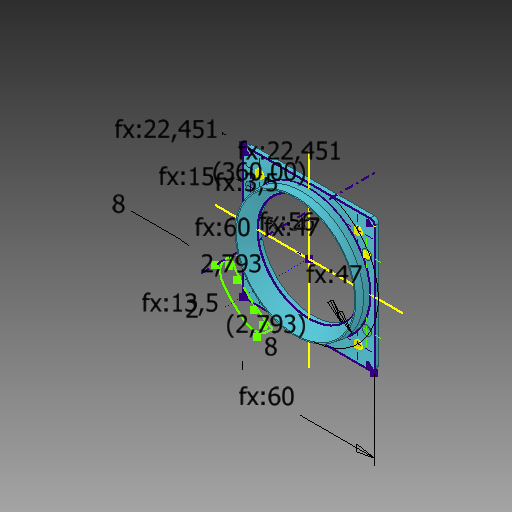
# Autodesk Inventor part: Front Ring
Saved by Autodesk Inventor 2019 (Build 230136000, 136)
## iProperties
Created: 2018-04-26
Part Number: Front Ring
Material: Generic
Document SubType Name: Modeling
Designer: Frank
Density: 1 g/cm^3
Appearance: Cadet Blue
Mass: 6.14957 g
Surface Area: 75.0161 cm^2
Volume: 6.14957 cm^3
RuleStatus: InUse
AfterAnyParamChange0: 1-RuleEncoderRight
Author: Frank
Autodesk Inventor part; units mm, degrees
ref_plane "YZ Plane" through (0, 0, 0) normal (1, 0, 0) x (0, 1, 0)
ref_plane "XZ Plane" through (0, 0, 0) normal (0, 1, 0) x (-1, 0, 0)
ref_plane "XY Plane" through (0, 0, 0) normal (0, 0, 1) x (1, 0, 0)
sketch "Sketch1" plane through (0, 0, 0) normal (0, 0, 1) x (1, 0, 0)
  circle A0 centre (0, 0) radius 28
  circle A1 centre (0, 0) radius 23.5
  line L0 (0, -39.2) -> (0, 39.2) projected
  line L1 (-39.2, 0) -> (39.2, 0) projected
  dimension "d0" = 56
  dimension "d1" = 47
  constraints: 2 centre point, 2 coincident
  measures "d0" diameter of A0
  measures "d1" diameter of A1
extrude "Extrusion1" add sketch "Sketch1" along normal blind 6 contours L1 A1 L0 A0 | A0 L0 A1 L1 | L0 A1 L1 A0 | A0 L1 A1 L0
chamfer "Chamfer1" distance 0.5 distance2 3 1 edges at (-28, 0, 6) measured on face at (-27.5, 0, 6)
chamfer "Chamfer2" distance 3.5 distance2 6 1 edges at (-23.5, 0, 6) measured on face at (-24, 0, 6)
sketch "Sketch3" plane through (0, 0, 0) normal (0, 0, -1) x (-1, 0, 0)
  line L0 (28, -30) -> (-28, -30)
  line L1 (-30, -28) -> (-30, 28)
  line L2 (-28, 30) -> (28, 30)
  line L3 (30, 28) -> (30, -28)
  circle A0 centre (0, 0) radius 23.5
  arc A1 (28, -30) -> (30, -28) centre (28, -28) ccw
  arc A2 (30, 28) -> (28, 30) centre (28, 28) ccw
  arc A3 (-30, -28) -> (-28, -30) centre (-28, -28) ccw
  arc A4 (-28, 30) -> (-30, 28) centre (-28, 28) ccw
  line L4 (0, -42.5799) -> (0, 42.5799) projected
  line L5 (42.5799, 0) -> (-42.5799, 0) projected
  point P0 (30, -30)
  point P1 (-30, -30)
  point P2 (30, 30)
  point P3 (26.5, 15)
  point P4 (26.5, 15)
  point P5 (22.4506, 22.4506)
  point P6 (-22.4506, 22.4506)
  point P7 (-22.4506, -22.4506)
  point P8 (22.4506, -22.4506)
  point P9 (-26.5, -15)
  point P10 (-26.5, 15)
  point P11 (26.5, -15)
  dimension "d19" = 60
  dimension "d20" = 60
  dimension "d23" = 47
  dimension "d24" = 2
  dimension "d40" = 3.5
  dimension "d50" = 15
  dimension "d54" = 22.4506
  dimension "d55" = 22.4506
  dimension "d58" = 360
  constraints: 8 end point, 8 point on circle, 8 tangent, 6 point on line, 5 centre point, 4 coincident, 3 equal radius, 2 parallel, 1 horizontal, 1 perpendicular, 9 other
  measures "d19" distance of point (30, 30) point (30, -30)
  measures "d20" distance of point (30, -30) point (-30, -30)
  measures "d23" diameter of A0
  measures "d24" radius of A1
  measures "d40" distance from line of point (26.5, 15) L3
  measures "d50" distance from line of L5 point (26.5, 15)
  measures "d54" horizontal distance of point (0, 0) point (22.451, 22.451)
  measures "d55" distance from line of L4 point (22.451, 22.451)
extrude "Extrusion3" add sketch "Sketch3" along normal blind 2 separate body contours L0 L4 A0 L5 L3 A1 | L0 A3 L1 L5 A0 L4 | L5 A0 L4 L2 A2 L3 | L5 L1 A4 L2 L4 A0
hole "Hole2" at (22.4506, 22.4506, 0) at (-22.4506, 22.4506, 0) direction (0, 0, -1) diameter 3.4 end through all bodies 1 2 clearance for "Countersunk Flat Head Screw DIN EN ISO 2009" size "M3" standard "DIN"
hole "Hole3" at (-26.5, 15, 0) at (26.5, 15, 0) direction (0, 0, -1) diameter 2.4 end through all countersink diameter 4.4 countersink angle 90 bodies 2 clearance for "Countersunk Flat Head Screw DIN EN ISO 2009" size "M2" standard "DIN"
hole "Hole4" at (22.4506, -22.4506, 0) direction (0, 0, -1) diameter 3.4 end through all bodies 1 2 clearance for "Countersunk Flat Head Screw DIN EN ISO 2009" size "M3" standard "DIN"
hole "Hole5" at (-22.4506, -22.4506, 0) direction (0, 0, -1) diameter 3.4 end through all bodies 1 2 clearance for "Countersunk Flat Head Screw DIN EN ISO 2009" size "M3" standard "DIN"
sketch "Sketch5" plane through (0, 0, 0) normal (0, 0, 1) x (1, 0, 0)
  arc A0 (-34.6205, -34.676) -> (-29.6559, -39.0068) centre (0, 0) ccw
  line L0 (0, 0) -> (-39.3527, -39.4158) construction
  line L1 (-49.0286, -30) -> (30, 49.1553)
  arc A1 (-35.7814, -16.7315) -> (-16.6742, -35.8081) centre (0, 0) ccw
  arc A2 (-38.9592, -29.7183) -> (-34.6205, -34.676) centre (0, 0) ccw
  arc A3 (-38.2599, -19.214) -> (-38.9592, -29.7183) centre (-32.5985, -24.8664) ccw
  arc A4 (-29.6559, -39.0068) -> (-19.1527, -38.2906) centre (-24.8141, -32.6383) ccw
  arc A5 (-27.9083, -27.9531) -> (-16.6742, -35.8081) centre (0, 0) ccw
  line L2 (-19.1527, -38.2906) -> (-16.6742, -35.8081)
  line L3 (-19.1527, -38.2906) -> (-16.6742, -35.8081)
  circle A6 centre (-22.4506, -22.4506) radius 1.7 projected
  circle A7 centre (22.4506, -22.4506) radius 1.7 projected
  circle A8 centre (26.5, 15) radius 1.2 projected
  circle A9 centre (22.4506, 22.4506) radius 1.7 projected
  circle A10 centre (-22.4506, 22.4506) radius 1.7 projected
  circle A11 centre (0, 0) radius 23.5 projected
  line L4 (28, -30) -> (-28, -30) projected
  arc A12 (-30, -28) -> (-28, -30) centre (-28, -28) ccw projected
  line L5 (-30, -28) -> (-30, 28) projected
  arc A13 (-28, 30) -> (-30, 28) centre (-28, 28) ccw projected
  line L6 (-28, 30) -> (28, 30) projected
  arc A14 (30, 28) -> (28, 30) centre (28, 28) ccw projected
  line L7 (30, 28) -> (30, -28) projected
  arc A15 (28, -30) -> (30, -28) centre (28, -28) ccw projected
  line L8 (-38.2599, -19.214) -> (-35.7814, -16.7315)
  circle A16 centre (-36.5057, -20.753) radius 1.3964
  circle A17 centre (-20.75, -36.4975) radius 1.3964
  point P0 (-42.8342, -23.7956)
  point P1 (-23.727, -42.8722)
  dimension "d99" = 13.5
  dimension "d102" = 8
  dimension "d103" = 8
  dimension "d148" = 2.7928
  dimension "d149" = 2.7928
  constraints: 15 point on circle, 10 end point, 8 centre point, 6 point on line, 5 tangent, 4 coincident, 2 parallel, 1 collinear, 1 equal radius, 1 other
  measures "d99" distance from line of L0 point (-42.834, -23.796)
  measures "d102" radius of A3
  measures "d103" radius of A4
  measures "d148" diameter of A16
  measures "d149" diameter of A17
extrude "Extrusion5" [suppressed]
hole "Hole7" at (26.5, -15, 0) at (-26.5, -15, 0) direction (0, 0, -1) diameter 2.4 end through all bodies 1 2 clearance for "Countersunk Flat Head Screw DIN EN ISO 2009" size "M2" standard "DIN"
hole "Hole10" [suppressed]
chamfer "Chamfer7" [suppressed]
chamfer "Chamfer8" distance 1 angle 45 1 edges at (26.5, -13.8, 0)
chamfer "Chamfer9" distance 1 angle 45 1 edges at (-26.5, -13.8, 0)
pattern_circular "Circular Pattern2" [suppressed]
equation "\"d0\" = circle_dimension"
equation "\"d1\" = circle_dimension_inner"
equation "\"d2\" = ring_depth"
equation "\"d4\" = ring_outer_bevel_depth"
equation "\"d5\" = ring_outer_bevel_height"
equation "\"d7\" = ring_inner_bevel_depth"
equation "\"d8\" = ring_depth"
equation "\"d19\" = backplate_width"
equation "\"d20\" = backplate_width"
equation "\"d23\" = circle_dimension_inner"
equation "\"d40\" = screw_distance_outside"
equation "\"d50\" = screw_distance_center"
equation "\"d54\" = hole_distance"
equation "\"d55\" = hole_distance"
equation "\"d25\" = front_plate_thickness"
equation "\"d99\" = 0.5 * encoder_width"
equation "\"ring_depth\" = 6"
equation "\"backplate_width\" = 60"
equation "\"circle_dimension\" = 56"
equation "\"hole_distance\" = 22.45064"
equation "\"screw_distance_center\" = 15"
equation "\"screw_distance_outside\" = 3.5"
equation "\"hole_from_center\" = 63.5"
equation "\"ring_thickness\" = 9"
equation "\"ring_outer_bevel_height\" = 3"
equation "\"ring_outer_bevel_depth\" = 0.5"
equation "\"ring_inner_bevel_depth\" = 3.5"
equation "\"encoders\" = 0"
equation "\"front_plate_thickness\" = 2"
equation "\"glass_thickness\" = 2"
equation "\"ring_top_thickness\" = 2"
equation "\"circle_dimension_inner\" = 47"
equation "\"encoder_rad\" = 49"
equation "\"encoder_emboss\" = 0"
equation "\"encoder_width\" = 27"
equation "\"encoder_axis\" = 8"
equation "\"d124\" = 27"
equation "\"encoder_extrude_hight\" = 3"
equation "\"pointer_axis\" = 1"
equation "\"pointer_length\" = 18"
equation "\"pointer_axis_outside\" = 3"
body "Solid1"
body "Solid2"
body "Solid5"
